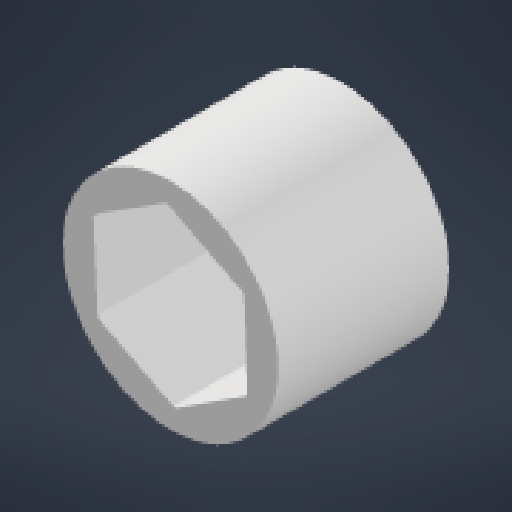
# Autodesk Inventor part: Power_Transmission_Space_Two
Saved by Autodesk Inventor 2024.2 (Build 282272000, 272)
## iProperties
Created: 2024-03-30
Part Number: Power_Transmission_Space_Two
Material: Generic
Document SubType Name: Modeling
Designer: warm
Density: 1 g/cm^3
Appearance: Default
Author: warm
Autodesk Inventor part; units mm, degrees
ref_plane "YZ Plane" through (0, 0, 0) normal (1, 0, 0) x (0, 1, 0)
ref_plane "XZ Plane" through (0, 0, 0) normal (0, 1, 0) x (-1, 0, 0)
sketch "Sketch1" plane through (0, 0, 0) normal (0, 0, 1) x (1, 0, 0)
  line L0 (0.1182, -3.9983) -> (-3.3246, -2.2242)
  arc A0 (-3.4035, -2.1015) -> (-3.3246, -2.2242) centre (0, 0) ccw
  line L1 (-3.4035, -2.1015) -> (-3.5885, 1.7671)
  arc A1 (-3.5217, 1.8967) -> (-3.5885, 1.7671) centre (0, 0) ccw
  line L2 (-3.5217, 1.8967) -> (-0.264, 3.9913)
  arc A2 (-0.1182, 3.9983) -> (-0.264, 3.9913) centre (0, 0) ccw
  line L3 (-0.1182, 3.9983) -> (3.3246, 2.2242)
  arc A3 (3.4035, 2.1015) -> (3.3246, 2.2242) centre (0, 0) ccw
  line L4 (3.4035, 2.1015) -> (3.5885, -1.7671)
  arc A4 (3.5217, -1.8967) -> (3.5885, -1.7671) centre (0, 0) ccw
  line L5 (3.5217, -1.8967) -> (0.264, -3.9913)
  arc A5 (0.1182, -3.9983) -> (0.264, -3.9913) centre (0, 0) ccw
  circle A6 centre (0, 0) radius 5
  point P0 (0, 0)
  dimension "d0" = 10
  constraints: 12 end point, 12 point on circle, 7 centre point, 1 coincident, 30 other
  measures "d0" diameter of A6
ref_plane "Work Plane1" through (-10.3993, -10.3993, 7.9391) normal (0, 0, -1) x (0.4581, 0.8889, 0)
extrude "Extrusion1" add sketch "Sketch1" along normal up to surface (7.9391 mm away)
body "Solid1"
